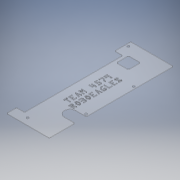
# Autodesk Inventor part: electronicsShield
Saved by Autodesk Inventor 2017 (Build 210142000, 142)
## iProperties
Created: 2017-02-18
Part Number: electronicsShield
Material: Generic
Document SubType Name: Sheet Metal
Designer: kingb
Density: 1 g/cm^3
Sheet Metal Rule: Default
Appearance: Clear - Light
Author: kingb
Autodesk Inventor part; units mm, degrees
(part 1 of 2)
ref_plane "YZ Plane" through (0, 0, 0) normal (1, 0, 0) x (0, 1, 0)
ref_plane "XZ Plane" through (0, 0, 0) normal (0, 1, 0) x (-1, 0, 0)
sketch "Sketch1" plane through (0, 0, 0) normal (0, 1, 0) x (-1, 0, 0)
  line L0 (0, 0) -> (203.2, 0)
  line L1 (203.2, -590.55) -> (0, -590.55)
  line L2 (0, -590.55) -> (0, 0)
  line L3 (203.2, 0) -> (165.1, 0)
  line L4 (165.1, -47.625) -> (203.2, -47.625)
  line L5 (203.2, -47.625) -> (203.2, 0)
  line L6 (203.2, -590.55) -> (165.1, -590.55)
  line L7 (165.1, -514.35) -> (203.2, -514.35)
  line L8 (203.2, -514.35) -> (203.2, -590.55)
  line L9 (165.1, -514.35) -> (165.1, -47.625)
  line L10 (203.2, 0) -> (203.2, -47.625)
  line L11 (203.2, -514.35) -> (203.2, -590.55)
  circle A0 centre (189.7062, -545.3062) radius 5.5563
  circle A1 centre (11.9063, -413.5437) radius 5.5563
  circle A2 centre (11.9063, -186.5312) radius 5.5563
  circle A3 centre (135.7313, -11.9062) radius 5.5562
  line L12 (189.7062, -590.55) -> (189.7062, -550.8625)
  line L13 (189.7062, -590.55) -> (229.3937, -590.55) construction
  line L14 (203.2, -545.3062) -> (195.2625, -545.3062)
  line L15 (0, -413.5437) -> (17.4625, -413.5437)
  line L16 (11.9063, -407.9875) -> (11.9063, -590.55)
  line L17 (0, -186.5312) -> (17.4625, -186.5312)
  line L18 (11.9063, -180.975) -> (11.9062, 0)
  line L19 (135.7312, 0) -> (135.7312, -6.35)
  line L20 (203.2, -11.9062) -> (141.2875, -11.9062)
  dimension "d0" = 203.2
  dimension "d1" = 590.55
  dimension "d2" = 38.1
  dimension "d3" = 47.625
  dimension "d4" = 38.1
  dimension "d5" = 76.2
  dimension "d6" = 165.1
  dimension "d7" = 11.1125
  dimension "d8" = 11.1125
  dimension "d9" = 11.1125
  dimension "d10" = 11.1125
  dimension "d11" = 39.6875
  dimension "d12" = 90
  dimension "d13" = 7.9375
  dimension "d14" = 17.4625
  dimension "d15" = 182.5625
  dimension "d16" = 17.4625
  dimension "d17" = 180.975
  dimension "d18" = 6.35
  dimension "d19" = 61.9125
  constraints: 42 end point, 8 line through centre, 8 point on circle, 8 point on line, 7 perpendicular, 6 horizontal, 5 parallel, 4 centre point, 2 vertical
  measures "d0" distance of L1.start L1.end
  measures "d1" distance of L0.end L1.start
  measures "d2" distance of L4.end L4.start
  measures "d3" distance of L4.start L3.end
  measures "d4" distance of L7.start L7.end
  measures "d5" distance of L6.end L7.start
  measures "d6" distance between parallel lines of L2 L9
  measures "d7" diameter of A0
  measures "d8" diameter of A1
  measures "d9" diameter of A2
  measures "d10" diameter of A3
  measures "d11" distance of L12.start L12.end
  measures "d12" angle of L13 L12
  measures "d13" distance of L14.start L14.end
  measures "d14" distance of L15.start L15.end
  measures "d15" distance of L16.start L16.end
  measures "d16" distance of L17.start L17.end
  measures "d17" distance of L18.start L18.end
  measures "d18" distance of L19.start L19.end
  measures "d19" distance of L20.start L20.end
extrude "Plate1" add sketch "Sketch1" along normal blind 3.048
extrude "Extrusion1" cut sketch "Sketch1" along normal up to next contours A2 L17 | L17 A2 | A3 | L15 L16 A1 | A1 L16 L15 | A1 L15 L16 | L16 L15 A1 | A0
sketch "Sketch2" plane through (0, 3.048, 0) normal (0, 1, 0) x (1, 0, 0)
  line L0 (-124.6492, 158.7906) -> (-124.6492, 431.7594) construction
  line L1 (-124.6492, 431.7594) -> (-53.1508, 431.7594) construction
  line L2 (-53.1508, 431.7594) -> (-53.1508, 158.7906) construction
  line L3 (-53.1508, 158.7906) -> (-124.6492, 158.7906) construction
  line L4 (-124.6492, 295.275) -> (-53.1508, 295.275) construction
  line L5 (0, 0) -> (-203.2, 0) construction
  line L6 (-88.9, 158.7906) -> (-88.9, 431.7594) construction
  line L7 (0, 590.55) -> (0, 0) construction
  spline S0 degree 2 poles (-120.1681, 207.8722) (-119.5073, 207.8722) (-118.6193, 206.9222) (-118.6193, 206.1995) knots 0 0 0 1 2 2 2
  spline S1 degree 2 poles (-118.6193, 206.1995) (-118.6193, 204.7126) (-120.4985, 204.7126) knots 0 0 0 1 1 1
  spline S2 degree 2 poles (-120.4985, 204.7126) (-120.8289, 204.7126) (-121.1799, 204.7126) knots 0 0 0 1 1 1
  spline S3 degree 2 poles (-121.1799, 204.7126) (-121.3451, 204.5887) (-121.3451, 203.3704) knots 0 0 0 1 1 1
  spline S4 degree 2 poles (-121.3451, 203.3704) (-121.3451, 202.5856) (-121.3038, 201.326) knots 0 0 0 1 1 1
  line L8 (-121.3038, 201.326) -> (-100.5295, 201.326)
  spline S5 degree 2 poles (-100.5295, 201.326) (-100.0133, 201.326) (-99.2079, 200.1695) (-99.2079, 199.6533) knots 0 0 0 1 2 2 2
  spline S6 degree 2 poles (-99.2079, 199.6533) (-99.2079, 199.0957) (-100.1991, 197.9806) (-100.7567, 197.9806) knots 0 0 0 1 2 2 2
  line L9 (-100.7567, 197.9806) -> (-121.3451, 197.9806)
  line L10 (-121.3451, 197.9806) -> (-121.3451, 194.8624)
  spline S7 degree 2 poles (-121.3451, 194.8624) (-120.4778, 194.7591) (-119.6105, 194.6352) knots 0 0 0 1 1 1
  spline S8 degree 2 poles (-119.6105, 194.6352) (-118.6193, 194.4287) (-118.6193, 193.1484) knots 0 0 0 1 1 1
  spline S9 degree 2 poles (-118.6193, 193.1484) (-118.6193, 192.6322) (-119.3834, 191.5583) (-119.8583, 191.5583) knots 0 0 0 1 2 2 2
  line L11 (-119.8583, 191.5583) -> (-124.6079, 191.5583)
  line L12 (-124.6079, 191.5583) -> (-124.6079, 207.8722)
  line L13 (-124.6079, 207.8722) -> (-120.1681, 207.8722)
  spline S10 degree 2 poles (-100.8806, 231.6821) (-100.2817, 231.6821) (-99.2079, 230.6909) (-99.2079, 230.1333) knots 0 0 0 1 2 2 2
  line L14 (-99.2079, 230.1333) -> (-99.2079, 215.4922)
  line L15 (-99.2079, 215.4922) -> (-124.6079, 215.4922)
  line L16 (-124.6079, 215.4922) -> (-124.6079, 230.2572)
  spline S11 degree 2 poles (-124.6079, 230.2572) (-124.6079, 230.7735) (-123.5341, 231.6821) (-122.9972, 231.6821) knots 0 0 0 1 2 2 2
  spline S12 degree 2 poles (-122.9972, 231.6821) (-122.4809, 231.6821) (-121.3658, 230.5669) (-121.3658, 230.0507) knots 0 0 0 1 2 2 2
  line L17 (-121.3658, 230.0507) -> (-121.3658, 218.7136)
  line L18 (-121.3658, 218.7136) -> (-113.5599, 218.7136)
  line L19 (-113.5599, 218.7136) -> (-113.5599, 224.0208)
  spline S13 degree 2 poles (-113.5599, 224.0208) (-113.5599, 224.5783) (-112.5687, 225.2598) (-111.9699, 225.2598) knots 0 0 0 1 2 2 2
  spline S14 degree 2 poles (-111.9699, 225.2598) (-111.3916, 225.2598) (-110.3591, 224.537) (-110.3591, 224.0208) knots 0 0 0 1 2 2 2
  line L20 (-110.3591, 224.0208) -> (-110.3591, 218.7136)
  line L21 (-110.3591, 218.7136) -> (-102.512, 218.7136)
  line L22 (-102.512, 218.7136) -> (-102.512, 230.1333)
  spline S15 degree 2 poles (-102.512, 230.1333) (-102.512, 230.6909) (-101.4381, 231.6821) (-100.8806, 231.6821) knots 0 0 0 1 2 2 2
  spline S16 degree 2 poles (-100.798, 255.6159) (-99.2079, 255.6159) (-99.2079, 254.0258) knots 0 0 0 1 1 1
  spline S17 degree 2 poles (-99.2079, 254.0258) (-99.2079, 253.0759) (-100.6741, 252.4357) knots 0 0 0 1 1 1
  spline S18 degree 2 poles (-100.6741, 252.4357) (-102.037, 252.0021) (-104.7422, 251.0728) knots 0 0 0 1 1 1
  line L23 (-104.7422, 251.0728) -> (-104.7422, 244.0104)
  spline S19 degree 2 poles (-104.7422, 244.0104) (-103.0695, 243.5354) (-101.4381, 243.1017) knots 0 0 0 1 1 1
  spline S20 degree 2 poles (-101.4381, 243.1017) (-99.2079, 242.2964) (-99.2079, 241.0161) knots 0 0 0 1 1 1
  spline S21 degree 2 poles (-99.2079, 241.0161) (-99.2079, 240.4585) (-100.2817, 239.426) (-100.8806, 239.426) knots 0 0 0 1 2 2 2
  spline S22 degree 2 poles (-100.8806, 239.426) (-101.5207, 239.426) (-111.4536, 242.4203) knots 0 0 0 1 1 1
  spline S23 degree 2 poles (-111.4536, 242.4203) (-120.8702, 245.2494) (-122.8939, 245.9722) knots 0 0 0 1 1 1
  spline S24 degree 2 poles (-122.8939, 245.9722) (-124.5666, 246.5297) (-124.6492, 247.6035) knots 0 0 0 1 1 1
  line L24 (-124.6492, 247.6035) -> (-124.5666, 247.6861)
  spline S25 degree 2 poles (-124.5666, 247.6861) (-124.5253, 248.6361) (-121.0973, 249.7925) (-111.2058, 252.7042) knots 0 0 0 1 2 2 2
  spline S26 degree 2 poles (-111.2058, 252.7042) (-101.1697, 255.6159) (-100.798, 255.6159) knots 0 0 0 1 1 1
  line L25 (-108.0463, 250.2468) -> (-118.516, 247.6448)
  line L26 (-118.516, 247.6448) -> (-108.0463, 244.9809)
  line L27 (-108.0463, 244.9809) -> (-108.0463, 250.2468)
  spline S27 degree 2 poles (-100.7154, 279.6736) (-100.1991, 279.6736) (-99.2079, 278.5172) (-99.2079, 277.9596) knots 0 0 0 1 2 2 2
  spline S28 degree 2 poles (-99.2079, 277.9596) (-99.2079, 277.3608) (-100.1578, 276.3695) (-100.7567, 276.3695) knots 0 0 0 1 2 2 2
  line L28 (-100.7567, 276.3695) -> (-119.9203, 276.3695)
  spline S29 degree 2 poles (-119.9203, 276.3695) (-118.5986, 275.337) (-115.9141, 273.4165) knots 0 0 0 1 1 1
  spline S30 degree 2 poles (-115.9141, 273.4165) (-115.6043, 273.21) (-115.563, 273.21) knots 0 0 0 1 1 1
  spline S31 degree 2 poles (-115.563, 273.21) (-115.3978, 273.21) (-115.2739, 273.21) knots 0 0 0 1 1 1
  spline S32 degree 2 poles (-115.2739, 273.21) (-113.0024, 273.21) (-113.0024, 271.4341) knots 0 0 0 1 1 1
  spline S33 degree 2 poles (-113.0024, 271.4341) (-113.0024, 270.1125) (-114.0762, 269.906) knots 0 0 0 1 1 1
  spline S34 degree 2 poles (-114.0762, 269.906) (-114.5718, 269.906) (-115.563, 269.7201) knots 0 0 0 1 1 1
  spline S35 degree 2 poles (-115.563, 269.7201) (-116.5542, 269.2245) (-117.9172, 268.2746) knots 0 0 0 1 1 1
  spline S36 degree 2 poles (-117.9172, 268.2746) (-119.0323, 267.4279) (-120.1474, 266.5813) knots 0 0 0 1 1 1
  line L29 (-120.1474, 266.5813) -> (-100.6534, 266.5813)
  spline S37 degree 2 poles (-100.6534, 266.5813) (-100.1165, 266.5813) (-99.2079, 265.5074) (-99.2079, 264.9499) knots 0 0 0 1 2 2 2
  spline S38 degree 2 poles (-99.2079, 264.9499) (-99.2079, 264.3923) (-100.0752, 263.3598) (-100.6534, 263.3598) knots 0 0 0 1 2 2 2
  line L30 (-100.6534, 263.3598) -> (-124.6079, 263.3598)
  line L31 (-124.6079, 263.3598) -> (-124.6079, 267.5931)
  line L32 (-124.6079, 267.5931) -> (-118.991, 271.4548)
  line L33 (-118.991, 271.4548) -> (-124.6079, 275.5642)
  line L34 (-124.6079, 275.5642) -> (-124.6079, 279.6736)
  line L35 (-124.6079, 279.6736) -> (-100.7154, 279.6736)
  spline S39 degree 2 poles (-108.9962, 326.5087) (-108.3147, 326.5087) (-107.9637, 326.0338) knots 0 0 0 1 1 1
  spline S40 degree 2 poles (-107.9637, 326.0338) (-107.7778, 325.8066) (-107.4268, 324.9187) knots 0 0 0 1 1 1
  line L36 (-107.4268, 324.9187) -> (-100.4056, 324.9187)
  spline S41 degree 2 poles (-100.4056, 324.9187) (-99.8481, 324.9187) (-99.2079, 323.8861) (-99.2079, 323.2873) knots 0 0 0 1 2 2 2
  spline S42 degree 2 poles (-99.2079, 323.2873) (-99.2079, 322.771) (-99.9307, 321.6972) (-100.4469, 321.6972) knots 0 0 0 1 2 2 2
  line L37 (-100.4469, 321.6972) -> (-107.4268, 321.6972)
  line L38 (-107.4268, 321.6972) -> (-107.4268, 312.0328)
  line L39 (-107.4268, 312.0328) -> (-123.3689, 312.0328)
  spline S43 degree 2 poles (-123.3689, 312.0328) (-124.6079, 312.0328) (-124.6079, 313.6435) knots 0 0 0 1 1 1
  spline S44 degree 2 poles (-124.6079, 313.6435) (-124.6079, 314.1598) (-123.8851, 315.2336) (-123.4102, 315.2336) knots 0 0 0 1 2 2 2
  line L40 (-123.4102, 315.2336) -> (-110.8134, 315.2336)
  line L41 (-110.8134, 315.2336) -> (-110.8134, 321.6972)
  line L42 (-110.8134, 321.6972) -> (-120.6224, 321.6972)
  spline S45 degree 2 poles (-120.6224, 321.6972) (-121.1386, 321.6972) (-121.8614, 322.771) (-121.8614, 323.2873) knots 0 0 0 1 2 2 2
  spline S46 degree 2 poles (-121.8614, 323.2873) (-121.8614, 323.8448) (-121.056, 324.9187) (-120.5398, 324.9187) knots 0 0 0 1 2 2 2
  line L43 (-120.5398, 324.9187) -> (-110.8134, 324.9187)
  spline S47 degree 2 poles (-110.8134, 324.9187) (-110.5037, 325.4762) (-109.8842, 326.5087) (-108.9962, 326.5087) knots 0 0 0 1 2 2 2
  spline S48 degree 2 poles (-101.9957, 351.3512) (-101.1697, 351.3512) (-99.2079, 349.3894) (-99.2079, 348.5221) knots 0 0 0 1 2 2 2
  line L44 (-99.2079, 348.5221) -> (-99.2079, 340.1793)
  spline S49 degree 2 poles (-99.2079, 340.1793) (-99.2079, 339.663) (-99.9307, 337.8665) knots 0 0 0 1 1 1
  spline S50 degree 2 poles (-99.9307, 337.8665) (-100.6121, 336.2351) (-101.2729, 335.1613) (-101.9957, 335.1613) knots 0 0 0 1 2 2 2
  spline S51 degree 2 poles (-101.9957, 335.1613) (-102.6359, 335.1613) (-103.9162, 336.0079) (-103.9162, 336.6274) knots 0 0 0 1 2 2 2
  spline S52 degree 2 poles (-103.9162, 336.6274) (-103.9162, 336.8752) (-102.512, 339.9935) (-102.512, 340.1793) knots 0 0 0 1 2 2 2
  line L45 (-102.512, 340.1793) -> (-102.512, 348.0471)
  line L46 (-102.512, 348.0471) -> (-110.2972, 348.0471)
  line L47 (-110.2972, 348.0471) -> (-110.2972, 338.3827)
  line L48 (-110.2972, 338.3827) -> (-124.6079, 338.3827)
  line L49 (-124.6079, 338.3827) -> (-124.6079, 349.9056)
  spline S53 degree 2 poles (-124.6079, 349.9056) (-124.6079, 350.5458) (-123.6373, 351.3512) (-122.9972, 351.3512) knots 0 0 0 1 2 2 2
  spline S54 degree 2 poles (-122.9972, 351.3512) (-122.4396, 351.3512) (-121.3658, 350.6697) (-121.3658, 350.1534) knots 0 0 0 1 2 2 2
  line L50 (-121.3658, 350.1534) -> (-121.3658, 341.6248)
  line L51 (-121.3658, 341.6248) -> (-113.5599, 341.6248)
  line L52 (-113.5599, 341.6248) -> (-113.5599, 348.7699)
  spline S55 degree 2 poles (-113.5599, 348.7699) (-113.5599, 349.472) (-111.5981, 351.3512) (-110.896, 351.3512) knots 0 0 0 1 2 2 2
  line L53 (-110.896, 351.3512) -> (-101.9957, 351.3512)
  spline S56 degree 2 poles (-114.6338, 375.4089) (-113.9316, 375.4089) (-111.4536, 372.5385) knots 0 0 0 1 1 1
  spline S57 degree 2 poles (-111.4536, 372.5385) (-109.8842, 370.7006) (-108.3354, 368.8627) knots 0 0 0 1 1 1
  line L54 (-108.3354, 368.8627) -> (-100.5295, 368.8627)
  spline S58 degree 2 poles (-100.5295, 368.8627) (-100.0133, 368.8627) (-99.2079, 367.7889) (-99.2079, 367.2726) knots 0 0 0 1 2 2 2
  spline S59 degree 2 poles (-99.2079, 367.2726) (-99.2079, 366.5912) (-100.1165, 365.5174) (-100.7567, 365.5174) knots 0 0 0 1 2 2 2
  line L55 (-100.7567, 365.5174) -> (-109.1407, 365.5174)
  spline S60 degree 2 poles (-109.1407, 365.5174) (-109.9255, 365.5174) (-112.3622, 368.3878) knots 0 0 0 1 1 1
  spline S61 degree 2 poles (-112.3622, 368.3878) (-113.911, 370.2256) (-115.4598, 372.1048) knots 0 0 0 1 1 1
  line L56 (-115.4598, 372.1048) -> (-121.3658, 372.1048)
  line L57 (-121.3658, 372.1048) -> (-121.3658, 362.3991)
  spline S62 degree 2 poles (-121.3658, 362.3991) (-120.5398, 362.0481) (-120.3333, 361.8416) knots 0 0 0 1 1 1
  spline S63 degree 2 poles (-120.3333, 361.8416) (-120.0235, 361.5318) (-120.0235, 360.7678) knots 0 0 0 1 1 1
  spline S64 degree 2 poles (-120.0235, 360.7678) (-120.0235, 359.0951) (-121.6549, 359.0951) knots 0 0 0 1 1 1
  spline S65 degree 2 poles (-121.6549, 359.0951) (-123.0591, 359.0951) (-123.5341, 359.219) knots 0 0 0 1 1 1
  spline S66 degree 2 poles (-123.5341, 359.219) (-124.6079, 359.5287) (-124.6079, 360.5406) knots 0 0 0 1 1 1
  line L58 (-124.6079, 360.5406) -> (-124.6079, 375.4089)
  line L59 (-124.6079, 375.4089) -> (-114.6338, 375.4089)
  spline S67 degree 2 poles (-100.4056, 399.1569) (-99.2079, 399.1569) (-99.2079, 396.7201) knots 0 0 0 1 1 1
  spline S68 degree 2 poles (-99.2079, 396.7201) (-99.2079, 394.3247) (-100.8806, 394.3247) knots 0 0 0 1 1 1
  spline S69 degree 2 poles (-100.8806, 394.3247) (-102.1196, 394.3247) (-102.2848, 394.6757) knots 0 0 0 1 1 1
  spline S70 degree 2 poles (-102.2848, 394.6757) (-102.4294, 395.3159) (-102.6359, 395.9148) knots 0 0 0 1 1 1
  line L60 (-102.6359, 395.9148) -> (-113.1263, 395.9148)
  line L61 (-113.1263, 395.9148) -> (-113.1263, 384.2679)
  spline S71 degree 2 poles (-113.1263, 384.2679) (-113.1263, 383.9788) (-114.0762, 383.0289) (-114.324, 383.0289) knots 0 0 0 1 2 2 2
  line L62 (-114.324, 383.0289) -> (-123.3689, 383.0289)
  spline S72 degree 2 poles (-123.3689, 383.0289) (-123.7406, 383.0289) (-124.6079, 384.144) (-124.6079, 384.4744) knots 0 0 0 1 2 2 2
  line L63 (-124.6079, 384.4744) -> (-124.6079, 397.67)
  spline S73 degree 2 poles (-124.6079, 397.67) (-124.6079, 398.0417) (-123.7612, 399.1569) (-123.4102, 399.1569) knots 0 0 0 1 2 2 2
  line L64 (-123.4102, 399.1569) -> (-100.4056, 399.1569)
  line L65 (-116.3684, 395.9148) -> (-121.3658, 395.9148)
  line L66 (-121.3658, 395.9148) -> (-121.3658, 386.2504)
  line L67 (-121.3658, 386.2504) -> (-116.3684, 386.2504)
  line L68 (-116.3684, 386.2504) -> (-116.3684, 395.9148)
  spline S74 degree 2 poles (-82.5154, 195.9052) (-76.5268, 195.9052) (-76.7746, 188.9874) knots 0 0 0 1 1 1
  line L69 (-76.7746, 188.9874) -> (-64.5289, 195.9052)
  spline S75 degree 2 poles (-64.5289, 195.9052) (-62.9388, 195.6161) (-62.9388, 194.1913) knots 0 0 0 1 1 1
  spline S76 degree 2 poles (-62.9388, 194.1913) (-62.9388, 193.9022) (-63.4964, 192.9109) (-63.7855, 192.7251) knots 0 0 0 1 2 2 2
  spline S77 degree 2 poles (-63.7855, 192.7251) (-65.169, 191.9197) (-67.9981, 190.2883) knots 0 0 0 1 1 1
  spline S78 degree 2 poles (-67.9981, 190.2883) (-73.5118, 187.0462) (-76.8572, 185.0225) knots 0 0 0 1 1 1
  line L70 (-76.8572, 185.0225) -> (-76.8572, 182.7922)
  line L71 (-76.8572, 182.7922) -> (-64.1365, 182.7922)
  spline S79 degree 2 poles (-64.1365, 182.7922) (-63.8061, 182.7922) (-62.9388, 181.5945) (-62.9388, 181.2022) knots 0 0 0 1 2 2 2
  spline S80 degree 2 poles (-62.9388, 181.2022) (-62.9388, 180.6239) (-63.8061, 179.5914) (-64.3843, 179.5914) knots 0 0 0 1 2 2 2
  line L72 (-64.3843, 179.5914) -> (-88.3388, 179.5914)
  line L73 (-88.3388, 179.5914) -> (-88.3388, 191.5893)
  spline S81 degree 2 poles (-88.3388, 191.5893) (-88.3388, 192.1882) (-87.9464, 192.9935) knots 0 0 0 1 1 1
  spline S82 degree 2 poles (-87.9464, 192.9935) (-86.5422, 195.9052) (-82.5154, 195.9052) knots 0 0 0 1 1 1
  spline S83 degree 2 poles (-83.0316, 192.6012) (-85.0967, 192.6012) (-85.0967, 190.9904) knots 0 0 0 1 1 1
  line L74 (-85.0967, 190.9904) -> (-85.0967, 182.7922)
  line L75 (-85.0967, 182.7922) -> (-80.0993, 182.7922)
  line L76 (-80.0993, 182.7922) -> (-80.0993, 190.9904)
  spline S84 degree 2 poles (-80.0993, 190.9904) (-80.0993, 192.1262) (-81.1318, 192.436) knots 0 0 0 1 1 1
  spline S85 degree 2 poles (-81.1318, 192.436) (-81.6068, 192.6012) (-83.0316, 192.6012) knots 0 0 0 1 1 1
  spline S86 degree 2 poles (-75.5768, 219.7152) (-73.9042, 219.7152) (-71.2403, 218.4348) knots 0 0 0 1 1 1
  spline S87 degree 2 poles (-71.2403, 218.4348) (-69.1133, 217.361) (-67.0069, 216.3285) knots 0 0 0 1 1 1
  spline S88 degree 2 poles (-67.0069, 216.3285) (-64.9419, 215.4405) (-64.0952, 214.6558) knots 0 0 0 1 1 1
  spline S89 degree 2 poles (-64.0952, 214.6558) (-62.9388, 213.5407) (-62.9388, 211.6202) knots 0 0 0 1 1 1
  spline S90 degree 2 poles (-62.9388, 211.6202) (-62.9388, 209.6997) (-64.2191, 208.502) knots 0 0 0 1 1 1
  spline S91 degree 2 poles (-64.2191, 208.502) (-64.7767, 207.9857) (-69.1546, 205.7968) knots 0 0 0 1 1 1
  spline S92 degree 2 poles (-69.1546, 205.7968) (-71.6739, 204.5165) (-72.2728, 204.2893) knots 0 0 0 1 1 1
  spline S93 degree 2 poles (-72.2728, 204.2893) (-74.0281, 203.5665) (-75.5768, 203.5252) knots 0 0 0 1 1 1
  line L77 (-75.5768, 203.5252) -> (-76.4648, 203.5252)
  spline S94 degree 2 poles (-76.4648, 203.5252) (-78.1375, 203.4839) (-84.6217, 207.0358) knots 0 0 0 1 1 1
  spline S95 degree 2 poles (-84.6217, 207.0358) (-86.6661, 208.1922) (-87.265, 208.7911) knots 0 0 0 1 1 1
  spline S96 degree 2 poles (-87.265, 208.7911) (-88.2562, 209.7823) (-88.3388, 211.5789) knots 0 0 0 1 1 1
  line L78 (-88.3388, 211.5789) -> (-88.3388, 211.9713)
  spline S97 degree 2 poles (-88.3388, 211.9713) (-88.4214, 213.8917) (-86.3357, 215.2547) knots 0 0 0 1 1 1
  spline S98 degree 2 poles (-86.3357, 215.2547) (-84.4359, 216.1633) (-82.5567, 217.1132) knots 0 0 0 1 1 1
  spline S99 degree 2 poles (-82.5567, 217.1132) (-80.884, 217.9599) (-79.2113, 218.8478) knots 0 0 0 1 1 1
  spline S100 degree 2 poles (-79.2113, 218.8478) (-77.1669, 219.7152) (-75.5768, 219.7152) knots 0 0 0 1 1 1
  spline S101 degree 2 poles (-75.6181, 216.4111) (-76.6094, 216.4111) (-77.2495, 216.122) knots 0 0 0 1 1 1
  spline S102 degree 2 poles (-77.2495, 216.122) (-79.0874, 215.3373) (-81.5448, 214.057) knots 0 0 0 1 1 1
  spline S103 degree 2 poles (-81.5448, 214.057) (-85.0967, 212.1778) (-85.0967, 211.6202) knots 0 0 0 1 1 1
  spline S104 degree 2 poles (-85.0967, 211.6202) (-85.0967, 211.0213) (-84.6217, 210.6909) knots 0 0 0 1 1 1
  spline S105 degree 2 poles (-84.6217, 210.6909) (-83.9403, 210.1747) (-81.1112, 208.8324) knots 0 0 0 1 1 1
  spline S106 degree 2 poles (-81.1112, 208.8324) (-78.5299, 207.5521) (-77.3734, 207.0978) knots 0 0 0 1 1 1
  spline S107 degree 2 poles (-77.3734, 207.0978) (-76.4029, 206.7467) (-75.6181, 206.7467) knots 0 0 0 1 1 1
  spline S108 degree 2 poles (-75.6181, 206.7467) (-74.7715, 206.7467) (-74.09, 206.9945) knots 0 0 0 1 1 1
  spline S109 degree 2 poles (-74.09, 206.9945) (-68.9894, 209.1009) (-66.4494, 210.8974) knots 0 0 0 1 1 1
  spline S110 degree 2 poles (-66.4494, 210.8974) (-66.2429, 211.0213) (-66.2429, 211.3311) knots 0 0 0 1 1 1
  spline S111 degree 2 poles (-66.2429, 211.3311) (-66.2429, 212.0952) (-66.532, 212.343) knots 0 0 0 1 1 1
  spline S112 degree 2 poles (-66.532, 212.343) (-66.9656, 212.694) (-70.1045, 214.2635) knots 0 0 0 1 1 1
  spline S113 degree 2 poles (-70.1045, 214.2635) (-73.0988, 215.7709) (-73.9661, 216.122) knots 0 0 0 1 1 1
  spline S114 degree 2 poles (-73.9661, 216.122) (-74.6476, 216.4111) (-75.6181, 216.4111) knots 0 0 0 1 1 1
  spline S115 degree 2 poles (-70.1871, 243.7729) (-68.9274, 243.7729) (-68.1634, 243.6077) knots 0 0 0 1 1 1
  spline S116 degree 2 poles (-68.1634, 243.6077) (-66.057, 243.174) (-64.5289, 241.5426) knots 0 0 0 1 1 1
  spline S117 degree 2 poles (-64.5289, 241.5426) (-62.9388, 239.7874) (-62.9388, 237.7017) knots 0 0 0 1 1 1
  line L79 (-62.9388, 237.7017) -> (-62.9388, 227.4591)
  line L80 (-62.9388, 227.4591) -> (-88.3388, 227.4591)
  line L81 (-88.3388, 227.4591) -> (-88.3388, 238.0734)
  spline S118 degree 2 poles (-88.3388, 238.0734) (-88.3388, 239.8287) (-84.8695, 243.4218) (-83.1142, 243.6077) knots 0 0 0 1 2 2 2
  spline S119 degree 2 poles (-83.1142, 243.6077) (-81.7513, 243.7729) (-81.1938, 243.7729) knots 0 0 0 1 1 1
  spline S120 degree 2 poles (-81.1938, 243.7729) (-77.8484, 243.7729) (-75.7421, 241.5839) knots 0 0 0 1 1 1
  spline S121 degree 2 poles (-75.7421, 241.5839) (-74.2965, 242.8643) (-72.025, 243.7729) (-70.1871, 243.7729) knots 0 0 0 1 2 2 2
  spline S122 degree 2 poles (-70.9099, 240.3449) (-71.9837, 240.3449) (-73.9455, 238.8581) (-73.9455, 237.8256) knots 0 0 0 1 2 2 2
  line L82 (-73.9455, 237.8256) -> (-73.9455, 230.6805)
  line L83 (-73.9455, 230.6805) -> (-66.2842, 230.6805)
  line L84 (-66.2842, 230.6805) -> (-66.2842, 237.7017)
  spline S123 degree 2 poles (-66.2842, 237.7017) (-66.2842, 238.7961) (-68.246, 240.3449) (-69.3611, 240.3449) knots 0 0 0 1 2 2 2
  line L85 (-69.3611, 240.3449) -> (-70.9099, 240.3449)
  spline S124 degree 2 poles (-81.9578, 240.3449) (-83.0316, 240.3449) (-85.0967, 238.6309) (-85.0967, 237.5984) knots 0 0 0 1 2 2 2
  line L86 (-85.0967, 237.5984) -> (-85.0967, 230.6805)
  line L87 (-85.0967, 230.6805) -> (-77.4147, 230.6805)
  line L88 (-77.4147, 230.6805) -> (-77.4147, 237.5984)
  spline S125 degree 2 poles (-77.4147, 237.5984) (-77.4147, 240.3449) (-81.9578, 240.3449) knots 0 0 0 1 1 1
  spline S126 degree 2 poles (-75.5768, 267.5828) (-73.9042, 267.5828) (-71.2403, 266.3025) knots 0 0 0 1 1 1
  spline S127 degree 2 poles (-71.2403, 266.3025) (-69.1133, 265.2287) (-67.0069, 264.1961) knots 0 0 0 1 1 1
  spline S128 degree 2 poles (-67.0069, 264.1961) (-64.9419, 263.3082) (-64.0952, 262.5235) knots 0 0 0 1 1 1
  spline S129 degree 2 poles (-64.0952, 262.5235) (-62.9388, 261.4083) (-62.9388, 259.4878) knots 0 0 0 1 1 1
  spline S130 degree 2 poles (-62.9388, 259.4878) (-62.9388, 257.5674) (-64.2191, 256.3696) knots 0 0 0 1 1 1
  spline S131 degree 2 poles (-64.2191, 256.3696) (-64.7767, 255.8534) (-69.1546, 253.6644) knots 0 0 0 1 1 1
  spline S132 degree 2 poles (-69.1546, 253.6644) (-71.6739, 252.3841) (-72.2728, 252.157) knots 0 0 0 1 1 1
  spline S133 degree 2 poles (-72.2728, 252.157) (-74.0281, 251.4342) (-75.5768, 251.3929) knots 0 0 0 1 1 1
  line L89 (-75.5768, 251.3929) -> (-76.4648, 251.3929)
  spline S134 degree 2 poles (-76.4648, 251.3929) (-78.1375, 251.3516) (-84.6217, 254.9035) knots 0 0 0 1 1 1
  spline S135 degree 2 poles (-84.6217, 254.9035) (-86.6661, 256.0599) (-87.265, 256.6587) knots 0 0 0 1 1 1
  spline S136 degree 2 poles (-87.265, 256.6587) (-88.2562, 257.65) (-88.3388, 259.4465) knots 0 0 0 1 1 1
  line L90 (-88.3388, 259.4465) -> (-88.3388, 259.8389)
  spline S137 degree 2 poles (-88.3388, 259.8389) (-88.4214, 261.7594) (-86.3357, 263.1223) knots 0 0 0 1 1 1
  spline S138 degree 2 poles (-86.3357, 263.1223) (-84.4359, 264.0309) (-82.5567, 264.9809) knots 0 0 0 1 1 1
  spline S139 degree 2 poles (-82.5567, 264.9809) (-80.884, 265.8275) (-79.2113, 266.7155) knots 0 0 0 1 1 1
  spline S140 degree 2 poles (-79.2113, 266.7155) (-77.1669, 267.5828) (-75.5768, 267.5828) knots 0 0 0 1 1 1
  spline S141 degree 2 poles (-75.6181, 264.2787) (-76.6094, 264.2787) (-77.2495, 263.9896) knots 0 0 0 1 1 1
  spline S142 degree 2 poles (-77.2495, 263.9896) (-79.0874, 263.2049) (-81.5448, 261.9246) knots 0 0 0 1 1 1
  spline S143 degree 2 poles (-81.5448, 261.9246) (-85.0967, 260.0454) (-85.0967, 259.4878) knots 0 0 0 1 1 1
  spline S144 degree 2 poles (-85.0967, 259.4878) (-85.0967, 258.889) (-84.6217, 258.5586) knots 0 0 0 1 1 1
  spline S145 degree 2 poles (-84.6217, 258.5586) (-83.9403, 258.0423) (-81.1112, 256.7) knots 0 0 0 1 1 1
  spline S146 degree 2 poles (-81.1112, 256.7) (-78.5299, 255.4197) (-77.3734, 254.9654) knots 0 0 0 1 1 1
  spline S147 degree 2 poles (-77.3734, 254.9654) (-76.4029, 254.6144) (-75.6181, 254.6144) knots 0 0 0 1 1 1
  spline S148 degree 2 poles (-75.6181, 254.6144) (-74.7715, 254.6144) (-74.09, 254.8622) knots 0 0 0 1 1 1
  spline S149 degree 2 poles (-74.09, 254.8622) (-68.9894, 256.9685) (-66.4494, 258.7651) knots 0 0 0 1 1 1
  spline S150 degree 2 poles (-66.4494, 258.7651) (-66.2429, 258.889) (-66.2429, 259.1987) knots 0 0 0 1 1 1
  spline S151 degree 2 poles (-66.2429, 259.1987) (-66.2429, 259.9628) (-66.532, 260.2106) knots 0 0 0 1 1 1
  spline S152 degree 2 poles (-66.532, 260.2106) (-66.9656, 260.5617) (-70.1045, 262.1311) knots 0 0 0 1 1 1
  spline S153 degree 2 poles (-70.1045, 262.1311) (-73.0988, 263.6386) (-73.9661, 263.9896) knots 0 0 0 1 1 1
  spline S154 degree 2 poles (-73.9661, 263.9896) (-74.6476, 264.2787) (-75.6181, 264.2787) knots 0 0 0 1 1 1
  spline S155 degree 2 poles (-64.6115, 291.5166) (-64.0126, 291.5166) (-62.9388, 290.5254) (-62.9388, 289.9678) knots 0 0 0 1 2 2 2
  line L91 (-62.9388, 289.9678) -> (-62.9388, 275.3267)
  line L92 (-62.9388, 275.3267) -> (-88.3388, 275.3267)
  line L93 (-88.3388, 275.3267) -> (-88.3388, 290.0917)
  spline S156 degree 2 poles (-88.3388, 290.0917) (-88.3388, 290.608) (-87.265, 291.5166) (-86.7281, 291.5166) knots 0 0 0 1 2 2 2
  spline S157 degree 2 poles (-86.7281, 291.5166) (-86.2118, 291.5166) (-85.0967, 290.4015) (-85.0967, 289.8852) knots 0 0 0 1 2 2 2
  line L94 (-85.0967, 289.8852) -> (-85.0967, 278.5482)
  line L95 (-85.0967, 278.5482) -> (-77.2908, 278.5482)
  line L96 (-77.2908, 278.5482) -> (-77.2908, 283.8553)
  spline S158 degree 2 poles (-77.2908, 283.8553) (-77.2908, 284.4129) (-76.2996, 285.0944) (-75.7007, 285.0944) knots 0 0 0 1 2 2 2
  spline S159 degree 2 poles (-75.7007, 285.0944) (-75.1225, 285.0944) (-74.09, 284.3716) (-74.09, 283.8553) knots 0 0 0 1 2 2 2
  line L97 (-74.09, 283.8553) -> (-74.09, 278.5482)
  line L98 (-74.09, 278.5482) -> (-66.2429, 278.5482)
  line L99 (-66.2429, 278.5482) -> (-66.2429, 289.9678)
  spline S160 degree 2 poles (-66.2429, 289.9678) (-66.2429, 290.5254) (-65.169, 291.5166) (-64.6115, 291.5166) knots 0 0 0 1 2 2 2
  spline S161 degree 2 poles (-64.5289, 315.4504) (-62.9388, 315.4504) (-62.9388, 313.8604) knots 0 0 0 1 1 1
  spline S162 degree 2 poles (-62.9388, 313.8604) (-62.9388, 312.9104) (-64.405, 312.2703) knots 0 0 0 1 1 1
  spline S163 degree 2 poles (-64.405, 312.2703) (-65.7679, 311.8366) (-68.4731, 310.9074) knots 0 0 0 1 1 1
  line L100 (-68.4731, 310.9074) -> (-68.4731, 303.8449)
  spline S164 degree 2 poles (-68.4731, 303.8449) (-66.8004, 303.37) (-65.169, 302.9363) knots 0 0 0 1 1 1
  spline S165 degree 2 poles (-65.169, 302.9363) (-62.9388, 302.1309) (-62.9388, 300.8506) knots 0 0 0 1 1 1
  spline S166 degree 2 poles (-62.9388, 300.8506) (-62.9388, 300.293) (-64.0126, 299.2605) (-64.6115, 299.2605) knots 0 0 0 1 2 2 2
  spline S167 degree 2 poles (-64.6115, 299.2605) (-65.2516, 299.2605) (-75.1845, 302.2548) knots 0 0 0 1 1 1
  spline S168 degree 2 poles (-75.1845, 302.2548) (-84.6011, 305.0839) (-86.6248, 305.8067) knots 0 0 0 1 1 1
  spline S169 degree 2 poles (-86.6248, 305.8067) (-88.2975, 306.3643) (-88.3801, 307.4381) knots 0 0 0 1 1 1
  line L101 (-88.3801, 307.4381) -> (-88.2975, 307.5207)
  spline S170 degree 2 poles (-88.2975, 307.5207) (-88.2562, 308.4706) (-84.8282, 309.627) (-74.9367, 312.5387) knots 0 0 0 1 2 2 2
  spline S171 degree 2 poles (-74.9367, 312.5387) (-64.9006, 315.4504) (-64.5289, 315.4504) knots 0 0 0 1 1 1
  line L102 (-71.7772, 310.0813) -> (-82.2469, 307.4794)
  line L103 (-82.2469, 307.4794) -> (-71.7772, 304.8155)
  line L104 (-71.7772, 304.8155) -> (-71.7772, 310.0813)
  spline S172 degree 2 poles (-86.79, 339.5082) (-85.138, 339.5082) (-85.138, 338.3104) knots 0 0 0 1 1 1
  line L105 (-85.138, 338.3104) -> (-85.138, 332.5696)
  spline S173 degree 2 poles (-85.138, 332.5696) (-85.138, 331.8469) (-78.1788, 326.4158) (-77.1463, 326.4158) knots 0 0 0 1 2 2 2
  line L106 (-77.1463, 326.4158) -> (-67.4406, 326.4158)
  spline S174 degree 2 poles (-67.4406, 326.4158) (-67.2754, 326.4158) (-66.3255, 327.3244) (-66.2842, 327.4896) knots 0 0 0 1 2 2 2
  spline S175 degree 2 poles (-66.2842, 327.4896) (-66.2016, 327.9646) (-66.2016, 333.3957) knots 0 0 0 1 1 1
  spline S176 degree 2 poles (-66.2016, 333.3957) (-66.2016, 334.7173) (-66.2842, 335.089) knots 0 0 0 1 1 1
  spline S177 degree 2 poles (-66.2842, 335.089) (-66.3668, 335.2748) (-67.0895, 336.0802) (-67.2341, 336.0802) knots 0 0 0 1 2 2 2
  line L107 (-67.2341, 336.0802) -> (-71.199, 336.0802)
  line L108 (-71.199, 336.0802) -> (-71.199, 332.5696)
  spline S178 degree 2 poles (-71.199, 332.5696) (-71.199, 332.0947) (-72.3554, 331.248) (-72.8716, 331.248) knots 0 0 0 1 2 2 2
  spline S179 degree 2 poles (-72.8716, 331.248) (-73.4705, 331.248) (-74.5443, 332.1153) (-74.5443, 332.6935) knots 0 0 0 1 2 2 2
  line L109 (-74.5443, 332.6935) -> (-74.5443, 339.3843)
  line L110 (-74.5443, 339.3843) -> (-67.1308, 339.3843)
  spline S180 degree 2 poles (-67.1308, 339.3843) (-65.6853, 339.3843) (-64.3843, 337.9387) knots 0 0 0 1 1 1
  spline S181 degree 2 poles (-64.3843, 337.9387) (-63.2279, 336.7617) (-63.0214, 335.2335) knots 0 0 0 1 1 1
  spline S182 degree 2 poles (-63.0214, 335.2335) (-62.9388, 334.7586) (-62.9388, 332.0947) knots 0 0 0 1 1 1
  spline S183 degree 2 poles (-62.9388, 332.0947) (-62.9388, 328.7287) (-63.0627, 326.8288) knots 0 0 0 1 1 1
  spline S184 degree 2 poles (-63.0627, 326.8288) (-63.1453, 325.7963) (-65.8918, 323.1943) (-66.9243, 323.1943) knots 0 0 0 1 2 2 2
  line L111 (-66.9243, 323.1943) -> (-77.8277, 323.1943)
  spline S185 degree 2 poles (-77.8277, 323.1943) (-79.4385, 323.1943) (-88.3388, 330.2981) (-88.3388, 331.7643) knots 0 0 0 1 2 2 2
  spline S186 degree 2 poles (-88.3388, 331.7643) (-88.3388, 332.6522) (-88.3388, 334.4075) knots 0 0 0 1 1 1
  spline S187 degree 2 poles (-88.3388, 334.4075) (-88.3388, 336.1628) (-88.3388, 337.0301) knots 0 0 0 1 1 1
  spline S188 degree 2 poles (-88.3388, 337.0301) (-88.3388, 339.5082) (-86.79, 339.5082) knots 0 0 0 1 1 1
  spline S189 degree 2 poles (-64.6115, 363.442) (-64.0952, 363.442) (-62.9388, 362.5334) (-62.9388, 362.0171) knots 0 0 0 1 2 2 2
  line L112 (-62.9388, 362.0171) -> (-62.9388, 347.1282)
  line L113 (-62.9388, 347.1282) -> (-87.0998, 347.1282)
  spline S190 degree 2 poles (-87.0998, 347.1282) (-88.3388, 347.1282) (-88.3388, 348.7389) knots 0 0 0 1 1 1
  spline S191 degree 2 poles (-88.3388, 348.7389) (-88.3388, 349.2552) (-87.616, 350.329) (-87.1411, 350.329) knots 0 0 0 1 2 2 2
  line L114 (-87.1411, 350.329) -> (-66.2429, 350.329)
  line L115 (-66.2429, 350.329) -> (-66.2429, 361.7693)
  spline S192 degree 2 poles (-66.2429, 361.7693) (-66.2429, 362.3682) (-65.2103, 363.442) (-64.6115, 363.442) knots 0 0 0 1 2 2 2
  spline S193 degree 2 poles (-64.6115, 387.2519) (-64.0126, 387.2519) (-62.9388, 386.2607) (-62.9388, 385.7031) knots 0 0 0 1 2 2 2
  line L116 (-62.9388, 385.7031) -> (-62.9388, 371.062)
  line L117 (-62.9388, 371.062) -> (-88.3388, 371.062)
  line L118 (-88.3388, 371.062) -> (-88.3388, 385.827)
  spline S194 degree 2 poles (-88.3388, 385.827) (-88.3388, 386.3433) (-87.265, 387.2519) (-86.7281, 387.2519) knots 0 0 0 1 2 2 2
  spline S195 degree 2 poles (-86.7281, 387.2519) (-86.2118, 387.2519) (-85.0967, 386.1368) (-85.0967, 385.6205) knots 0 0 0 1 2 2 2
  line L119 (-85.0967, 385.6205) -> (-85.0967, 374.2835)
  line L120 (-85.0967, 374.2835) -> (-77.2908, 374.2835)
  line L121 (-77.2908, 374.2835) -> (-77.2908, 379.5906)
  spline S196 degree 2 poles (-77.2908, 379.5906) (-77.2908, 380.1482) (-76.2996, 380.8296) (-75.7007, 380.8296) knots 0 0 0 1 2 2 2
  spline S197 degree 2 poles (-75.7007, 380.8296) (-75.1225, 380.8296) (-74.09, 380.1069) (-74.09, 379.5906) knots 0 0 0 1 2 2 2
  line L122 (-74.09, 379.5906) -> (-74.09, 374.2835)
  line L123 (-74.09, 374.2835) -> (-66.2429, 374.2835)
  line L124 (-66.2429, 374.2835) -> (-66.2429, 385.7031)
  spline S198 degree 2 poles (-66.2429, 385.7031) (-66.2429, 386.2607) (-65.169, 387.2519) (-64.6115, 387.2519) knots 0 0 0 1 2 2 2
  spline S199 degree 2 poles (-66.6146, 411.3096) (-65.4581, 411.3096) (-62.9388, 409.3891) (-62.9388, 408.274) knots 0 0 0 1 2 2 2
  line L125 (-62.9388, 408.274) -> (-62.9388, 398.7542)
  spline S200 degree 2 poles (-62.9388, 398.7542) (-62.9388, 397.3913) (-65.7679, 394.9958) (-67.1308, 394.9958) knots 0 0 0 1 2 2 2
  spline S201 degree 2 poles (-67.1308, 394.9958) (-69.0513, 394.9958) (-69.0513, 396.6685) knots 0 0 0 1 1 1
  spline S202 degree 2 poles (-69.0513, 396.6685) (-69.0513, 397.8249) (-66.2429, 398.4238) (-66.2429, 398.9813) knots 0 0 0 1 2 2 2
  line L126 (-66.2429, 398.9813) -> (-66.2429, 407.7991)
  spline S203 degree 2 poles (-66.2429, 407.7991) (-66.3255, 407.8817) (-66.4081, 407.8817) knots 0 0 0 1 1 1
  line L127 (-66.4081, 407.8817) -> (-66.5939, 407.8817)
  spline S204 degree 2 poles (-66.5939, 407.8817) (-66.883, 407.8817) (-74.1933, 402.1409) knots 0 0 0 1 1 1
  spline S205 degree 2 poles (-74.1933, 402.1409) (-82.3295, 395.7599) (-82.5154, 395.5947) knots 0 0 0 1 1 1
  spline S206 degree 2 poles (-82.5154, 395.5947) (-83.3621, 394.9958) (-84.6837, 394.9958) knots 0 0 0 1 1 1
  spline S207 degree 2 poles (-84.6837, 394.9958) (-85.9434, 394.9958) (-88.3388, 396.9163) (-88.3388, 398.1966) knots 0 0 0 1 2 2 2
  line L128 (-88.3388, 398.1966) -> (-88.3388, 407.448)
  spline S208 degree 2 poles (-88.3388, 407.448) (-88.3388, 408.8316) (-85.3858, 411.3096) (-83.9403, 411.3096) knots 0 0 0 1 2 2 2
  spline S209 degree 2 poles (-83.9403, 411.3096) (-83.3414, 411.3096) (-82.2263, 410.2358) (-82.2263, 409.5956) knots 0 0 0 1 2 2 2
  spline S210 degree 2 poles (-82.2263, 409.5956) (-82.2263, 408.5218) (-85.0347, 407.6339) (-84.9934, 406.8904) knots 0 0 0 1 2 2 2
  line L129 (-84.9934, 406.8904) -> (-84.9934, 398.2792)
  spline S211 degree 2 poles (-84.9934, 398.2792) (-84.9934, 398.1966) (-84.725, 398.2379) knots 0 0 0 1 1 1
  spline S212 degree 2 poles (-84.725, 398.2379) (-84.5598, 398.2379) (-77.2289, 403.9787) knots 0 0 0 1 1 1
  spline S213 degree 2 poles (-77.2289, 403.9787) (-69.3198, 410.1945) (-68.7622, 410.6075) knots 0 0 0 1 1 1
  spline S214 degree 2 poles (-68.7622, 410.6075) (-67.7297, 411.3096) (-66.6146, 411.3096) knots 0 0 0 1 1 1
  dimension "d23" = 136.4844
  dimension "d24" = 71.4984
  dimension "d25" = 272.9688
  dimension "d26" = 295.275
  dimension "d27" = 88.9
  constraints: 4 end point, 4 midpoint, 2 other
  measures "d23" distance between parallel lines of L3 L4
  measures "d24" distance between parallel lines of L2 L0
  measures "d25" distance between parallel lines of L1 L3
  measures "d26" distance between parallel lines of L5 L4
  measures "d27" distance between parallel lines of L7 L6
extrude "Extrusion2" cut sketch "Sketch2" against normal up to next